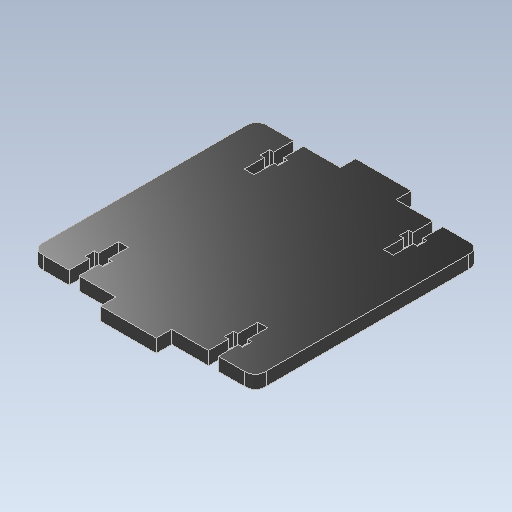
# Autodesk Inventor part: Mounting Base Bottom
Saved by Autodesk Inventor 2025 (Build 290162000, 162)
## iProperties
Created: 2024-05-30
Part Number: Mounting Base Bottom
Material: Polycarbonate, Smoke
Document SubType Name: Modeling
Designer: AlexForbes
Density: 1.2 g/cm^3
Appearance: Glossy - Black
Author: AlexForbes
Autodesk Inventor part; units mm, degrees
ref_plane "YZ Plane" through (0, 0, 0) normal (1, 0, 0) x (0, 1, 0)
ref_plane "XZ Plane" through (0, 0, 0) normal (0, 1, 0) x (-1, 0, 0)
sketch "Sketch1" plane through (0, 0, 0) normal (0, 1, 0) x (-1, 0, 0)
  line L0 (0, 0) -> (-101.6, 0)
  line L1 (-101.6, 0) -> (-101.6, -102.3)
  line L2 (-101.6, -102.3) -> (0, -102.3)
  line L3 (0, -102.3) -> (0, 0)
  dimension "d19" = 102.3
  dimension "d39" = 101.6
  constraints: 8 end point, 2 parallel, 1 horizontal, 1 perpendicular
  measures "d19" distance of L0.end L1.end
  measures "d39" distance of L1.end L2.end
extrude "Extrusion1" add sketch "Sketch1" along normal blind 6
ref_plane "Work Plane1" through (101.6, 0, -51.15) normal (0, 0, -1) x (-1, 0, 0)
sketch "Sketch3" plane through (0, 0, 0) normal (0, 1, 0) x (-1, 0, 0)
  line L0 (0, -102.3) -> (0, 0) projected
  line L1 (0, 0) -> (-101.6, 0) projected
  line L2 (-101.6, 0) -> (-101.6, -102.3) projected
  line L3 (-101.6, -102.3) -> (0, -102.3) projected
  line L4 (-38.1, -102.3) -> (-63.5, -102.3)
  line L5 (-63.5, -102.3) -> (-63.5, -109.3)
  line L6 (-63.5, -109.3) -> (-38.1, -109.3)
  line L7 (-38.1, -109.3) -> (-38.1, -102.3)
  line L8 (-101.6, -102.3) -> (0, -102.3) projected
  point P0 (-63.5, -102.3)
  point P1 (-50.8, -102.3)
  dimension "d20" = 7
  dimension "d31" = 25.4
  constraints: 8 end point, 2 midpoint, 2 parallel, 1 horizontal, 1 perpendicular, 1 point on line
  measures "d20" distance of L4.end L5.end
  measures "d31" distance of L5.end L6.end
extrude "Extrusion2" add sketch "Sketch3" along normal up to surface (6 mm away) contours L7 L6 L5 L3
mirror "Mirror1" about plane through (101.6, 0, -51.15) normal (0, 0, -1) of "Extrusion2"
sketch "Sketch4" plane through (0, 6, 0) normal (0, 1, 0) x (1, 0, 0)
  line L0 (14.925, 93.175) -> (14.925, 88.925)
  line L1 (23.175, 88.925) -> (23.175, 93.175)
  line L2 (16.8021, 79.8) -> (16.8021, 88.925)
  line L3 (16.8021, 93.175) -> (16.8021, 102.3)
  line L4 (21.2979, 102.3) -> (21.2979, 93.175)
  line L5 (21.2979, 88.925) -> (21.2979, 79.8)
  line L6 (23.175, 93.175) -> (21.2979, 93.175)
  line L7 (16.8021, 93.175) -> (14.925, 93.175)
  line L8 (14.925, 88.925) -> (16.8021, 88.925)
  line L9 (21.2979, 88.925) -> (23.175, 88.925)
  line L10 (16.8021, 79.8) -> (21.2979, 79.8)
  line L11 (16.8021, 102.3) -> (21.2979, 102.3)
  line L12 (80.3021, 93.175) -> (80.3021, 102.3)
  line L13 (78.425, 93.175) -> (78.425, 88.925)
  line L14 (80.3021, 79.8) -> (80.3021, 88.925)
  line L15 (86.675, 88.925) -> (86.675, 93.175)
  line L16 (78.425, 88.925) -> (80.3021, 88.925)
  line L17 (80.3021, 93.175) -> (78.425, 93.175)
  line L18 (84.7979, 88.925) -> (84.7979, 79.8)
  line L19 (84.7979, 102.3) -> (84.7979, 93.175)
  line L20 (86.675, 93.175) -> (84.7979, 93.175)
  line L21 (84.7979, 88.925) -> (86.675, 88.925)
  line L22 (80.3021, 79.8) -> (84.7979, 79.8)
  line L23 (80.3021, 102.3) -> (84.7979, 102.3)
  line L24 (38.1, 102.3) -> (0, 102.3) projected
  line L25 (101.6, 102.3) -> (63.5, 102.3) projected
  point P0 (0, 0)
  point P1 (19.05, 79.8)
  point P2 (82.55, 79.8)
  point P3 (19.05, 102.3)
  point P4 (82.55, 102.3)
  point P5 (82.55, 102.3)
  point P6 (19.05, 102.3)
  dimension "d25" = 4.25
  dimension "d26" = 8.25
  dimension "d28" = 4.4958
  dimension "d32" = 22.5
  constraints: 48 end point, 18 parallel, 12 equal length, 8 midpoint, 4 horizontal, 4 horizontal alignment, 4 perpendicular, 4 vertical, 2 vertical alignment
  measures "d25" distance of L1.end L1.start
  measures "d26" distance of L1.start L0.end
  measures "d28" distance between parallel lines of L4 L3
  measures "d32" distance between parallel lines of L10 L11
extrude "Extrusion3" cut sketch "Sketch4" against normal through all
fillet "Fillet1" radius 5 4 edges at (0, 3, 0) (101.6, 3, 0) (101.6, 3, -102.3) (0, 3, -102.3) curvature continuous yes
mirror "Mirror2" about plane through (101.6, 0, -51.15) normal (0, 0, -1) of "Extrusion3"
sketch "Sketch2" plane through (0, 6, 0) normal (0, 1, 0) x (1, 0, 0)
  line L0 (0, 0) -> (0, 6.7) construction
  line L1 (0, 6.7) -> (6.35, 6.7) construction
  line L2 (6.35, 6.7) -> (6.35, 0) construction
  line L3 (6.35, 0) -> (0, 0) construction
  dimension "d3" = 6.7
  dimension "d40" = 6.35
  constraints: 8 end point, 2 parallel, 1 coincident, 1 perpendicular, 1 vertical
  measures "d3" distance of L1.end L2.end
  measures "d40" distance of L0.end L1.end
hole "Hole1" [suppressed]
pattern_linear "Rectangular Pattern1" [suppressed]
body "Solid1"
